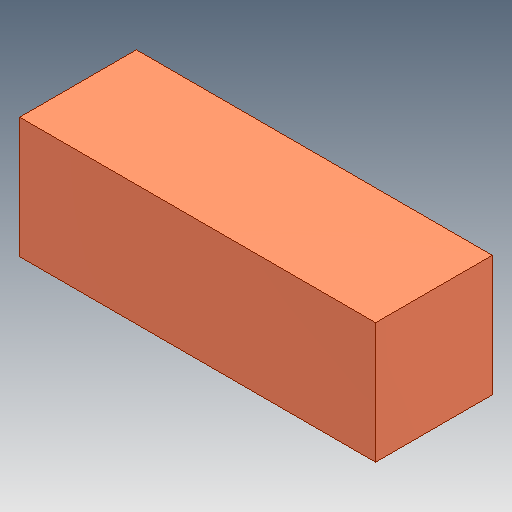
# Autodesk Inventor part: 4_7K
Saved by Autodesk Inventor 2017 (Build 210142000, 142)
## iProperties
Part Number: 4_7K
Material: Generisch
Document SubType Name: Modeling
Designer: Werkstatt
Density: 1 g/cm^3
Appearance: 0402-RES, 4_7K
Author: Werkstatt
Autodesk Inventor part; units mm, degrees
ref_plane "YZ Plane" through (0, 0, 0) normal (1, 0, 0) x (0, 1, 0)
ref_plane "XZ Plane" through (0, 0, 0) normal (0, 1, 0) x (-1, 0, 0)
ref_plane "XY Plane" through (0, 0, 0) normal (0, 0, 1) x (1, 0, 0)
sketch "0402-RES, 4_7K_47" plane through (0, 0, 0) normal (0, 0, 1) x (1, 0, 0)
  line L0 (-1.473, 0.483) -> (1.473, 0.483)
  line L1 (1.473, 0.483) -> (1.473, -0.483)
  line L2 (1.473, -0.483) -> (-1.473, -0.483)
  line L3 (-1.473, -0.483) -> (-1.473, 0.483)
  constraints: 8 end point
extrude "Extrusion1" add sketch "0402-RES, 4_7K_47" along normal blind 1
